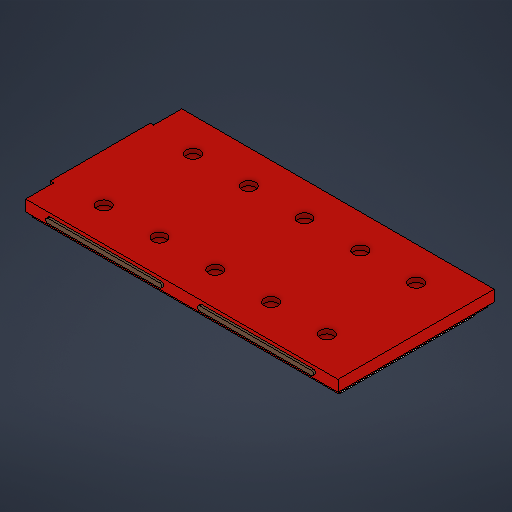
# Autodesk Inventor part: SACMI PH1500 30X60 DIE SET TOP
Saved by Autodesk Inventor 2025 (Build 290162000, 162)
## iProperties
Created: 2024-05-03
Part Number: SACMI PH1500 30X60 DIE SET TOP
Material: Generic
Document SubType Name: Modeling
Designer: zulet
Density: 1 g/cm^3
Appearance: Orange-Red
Author: zulet
Autodesk Inventor part; units mm, degrees
ref_plane "YZ Plane" through (0, 0, 0) normal (1, 0, 0) x (0, 1, 0)
ref_plane "XZ Plane" through (0, 0, 0) normal (0, 1, 0) x (-1, 0, 0)
ref_plane "XY Plane" through (0, 0, 0) normal (0, 0, 1) x (1, 0, 0)
sketch "Sketch1" plane through (0, 0, 0) normal (0, 1, 0) x (-1, 0, 0)
  line L0 (700, 350) -> (-700, 350)
  line L1 (-700, 350) -> (-700, -350)
  line L2 (-700, -350) -> (700, -350)
  line L3 (700, -350) -> (700, 350)
  line L4 (700, 350) -> (-700, -350) construction
  line L5 (-700, 350) -> (700, -350) construction
  point P0 (0, 0)
  dimension "d0" = 1400
  dimension "d1" = 700
  constraints: 12 end point, 2 midpoint, 2 parallel, 1 horizontal, 1 perpendicular
  measures "d0" distance of L2.end L1.end
  measures "d1" distance of L1.end L0.end
extrude "Extrusion1" add sketch "Sketch1" along normal blind 70
sketch "Sketch2" plane through (0, 70, 0) normal (0, 1, 0) x (1, 0, 0)
  line L0 (-500, -200) -> (500, -200) construction
  line L1 (500, -200) -> (500, 200) construction
  line L2 (500, 200) -> (-500, 200) construction
  line L3 (-500, 200) -> (-500, -200) construction
  line L4 (-500, -200) -> (500, 200) construction
  line L5 (500, -200) -> (-500, 200) construction
  circle A0 centre (500, -200) radius 30
  circle A1 centre (250, -200) radius 30
  circle A2 centre (0, -200) radius 30
  circle A3 centre (-250, -200) radius 30
  circle A4 centre (-500, -200) radius 30
  circle A5 centre (500, 200) radius 30
  circle A6 centre (250, 200) radius 30
  circle A7 centre (0, 200) radius 30
  circle A8 centre (-250, 200) radius 30
  circle A9 centre (-500, 200) radius 30
  point P0 (0, 0)
  dimension "d4" = 1000
  dimension "d5" = 400
  dimension "d6" = 60
  dimension "d9" = 250
  dimension "d12" = 400
  constraints: 12 end point, 10 centre point, 2 horizontal, 2 midpoint, 2 parallel, 1 coincident, 1 perpendicular, 1 vertical, 18 other
  measures "d4" distance of L2.end L1.end
  measures "d5" distance of L1.end L0.end
  measures "d6" diameter of A0
  measures "d9" distance of A0.centre A1.centre
  measures "d12" distance of A0.centre A5.centre
extrude "Extrusion2" cut sketch "Sketch2" against normal blind 20
sketch "Sketch3" plane through (0, 0, 0) normal (0, -1, 0) x (1, 0, 0)
  line L0 (700, 350) -> (700, -350) projected
  line L1 (-700, 350) -> (700, 350) projected
  line L2 (-700, -350) -> (-700, 350) projected
  line L3 (700, -350) -> (-700, -350) projected
  line L4 (-685, 335) -> (685, 335)
  line L5 (685, 335) -> (685, -335)
  line L6 (685, -335) -> (-685, -335)
  line L7 (-685, -335) -> (-685, 335)
  point P0 (0, 0)
  dimension "d17" = 15
  constraints: 8 end point, 3 other
  measures "d17" distance between parallel lines of L2 L7
extrude "Extrusion3" cut sketch "Sketch3" against normal blind 20
sketch "Sketch4" plane through (-700, 70, -350) normal (-1, 0, 0) x (0, 0, 1)
  line L0 (125, 0) -> (575, 0)
  line L1 (575, 0) -> (575, -70)
  line L2 (575, -70) -> (125, -70)
  line L3 (125, -70) -> (125, 0)
  line L4 (125, 0) -> (575, -70) construction
  line L5 (575, 0) -> (125, -70) construction
  line L6 (0, 0) -> (700, 0) projected
  line L7 (685, -70) -> (15, -70) projected
  line L8 (350, -35) -> (350, -70) construction
  dimension "d20" = 450
  constraints: 14 end point, 2 collinear, 2 midpoint, 2 parallel, 1 horizontal, 1 perpendicular, 1 vertical
  measures "d20" distance of L0.start L0.end
extrude "Extrusion4" add sketch "Sketch4" along normal blind 15 and the other way blind 15
sketch "Sketch5" plane through (0, 0, 0) normal (0, -1, 0) x (1, 0, 0)
  line L0 (-715, 225) -> (-715, -225) construction
  line L1 (-715, 0) -> (700, 0) construction
  line L2 (700, 350) -> (700, -350) construction
  line L3 (-660, 300) -> (-360, 300) construction
  line L4 (-360, 300) -> (-360, -300) construction
  line L5 (-360, -300) -> (-660, -300) construction
  line L6 (-660, -300) -> (-660, 300) construction
  line L7 (-660, 300) -> (-360, -300) construction
  line L8 (-360, 300) -> (-660, -300) construction
  line L9 (-370, 290) -> (-650, 290)
  line L10 (-650, 290) -> (-650, -290)
  line L11 (-650, -290) -> (-370, -290)
  line L12 (-370, -290) -> (-370, 290)
  line L13 (-320, 300) -> (-20, 300) construction
  line L14 (-20, 300) -> (-20, -300) construction
  line L15 (-20, -300) -> (-320, -300) construction
  line L16 (-320, -300) -> (-320, 300) construction
  line L17 (-320, 300) -> (-20, -300) construction
  line L18 (-20, 300) -> (-320, -300) construction
  line L19 (-30, 290) -> (-310, 290)
  line L20 (-310, 290) -> (-310, -290)
  line L21 (-310, -290) -> (-30, -290)
  line L22 (-30, -290) -> (-30, 290)
  line L23 (20, 300) -> (320, 300) construction
  line L24 (320, 300) -> (320, -300) construction
  line L25 (320, -300) -> (20, -300) construction
  line L26 (20, -300) -> (20, 300) construction
  line L27 (20, 300) -> (320, -300) construction
  line L28 (320, 300) -> (20, -300) construction
  line L29 (310, 290) -> (30, 290)
  line L30 (30, 290) -> (30, -290)
  line L31 (30, -290) -> (310, -290)
  line L32 (310, -290) -> (310, 290)
  line L33 (360, 300) -> (660, 300) construction
  line L34 (660, 300) -> (660, -300) construction
  line L35 (660, -300) -> (360, -300) construction
  line L36 (360, -300) -> (360, 300) construction
  line L37 (360, 300) -> (660, -300) construction
  line L38 (660, 300) -> (360, -300) construction
  line L39 (650, 290) -> (370, 290)
  line L40 (370, 290) -> (370, -290)
  line L41 (370, -290) -> (650, -290)
  line L42 (650, -290) -> (650, 290)
  line L43 (0, 0) -> (0, 331.4551) construction
  point P0 (-510, 0)
  point P1 (-170, 0)
  point P2 (170, 0)
  point P3 (510, 0)
  dimension "d25" = 300
  dimension "d26" = 600
  dimension "d27" = 10
  dimension "d30" = 340
  constraints: 84 end point, 5 parallel, 4 midpoint, 2 horizontal, 2 perpendicular, 1 point on line, 61 other
  measures "d25" distance of L4.end L5.end
  measures "d26" distance of L3.end L4.end
  measures "d27" distance between parallel lines of L3 L9
  measures "d30" distance of L3.start L13.start
extrude "Extrusion5" add sketch "Sketch5" along normal blind 20
sketch "Sketch6" plane through (0, -20, 0) normal (0, -1, 0) x (1, 0, 0)
  line L0 (-650, 290) -> (-650, -290) construction
  line L1 (-650, -290) -> (-370, -290) construction
  line L2 (-370, -290) -> (-370, 290) construction
  line L3 (-370, 290) -> (-650, 290) construction
  line L4 (-310, 290) -> (-310, -290) construction
  line L5 (-310, -290) -> (-30, -290) construction
  line L6 (-30, -290) -> (-30, 290) construction
  line L7 (-30, 290) -> (-310, 290) construction
  line L8 (30, 290) -> (30, -290) construction
  line L9 (30, -290) -> (310, -290) construction
  line L10 (310, -290) -> (310, 290) construction
  line L11 (310, 290) -> (30, 290) construction
  line L12 (370, 290) -> (370, -290) construction
  line L13 (370, -290) -> (650, -290) construction
  line L14 (650, -290) -> (650, 290) construction
  line L15 (650, 290) -> (370, 290) construction
  line L16 (-360, 300) -> (-360, -300)
  line L17 (-360, -300) -> (-660, -300)
  line L18 (-660, -300) -> (-660, 300)
  line L19 (-660, 300) -> (-360, 300)
  line L20 (-320, -300) -> (-320, 300)
  line L21 (-320, 300) -> (-20, 300)
  line L22 (-20, 300) -> (-20, -300)
  line L23 (-20, -300) -> (-320, -300)
  line L24 (20, -300) -> (20, 300)
  line L25 (20, 300) -> (320, 300)
  line L26 (320, 300) -> (320, -300)
  line L27 (320, -300) -> (20, -300)
  line L28 (360, -300) -> (360, 300)
  line L29 (360, 300) -> (660, 300)
  line L30 (660, 300) -> (660, -300)
  line L31 (660, -300) -> (360, -300)
  point P0 (0, 0)
  dimension "d37" = 10
  dimension "d38" = 10
  dimension "d39" = 10
  dimension "d40" = 10
  constraints: 32 end point, 12 other
  measures "d37" distance between parallel lines of L2 L16
  measures "d38" distance between parallel lines of L4 L20
  measures "d39" distance between parallel lines of L8 L24
  measures "d40" distance between parallel lines of L12 L28
extrude "Extrusion6" add sketch "Sketch6" along normal blind 10
sketch "Sketch7" plane through (-650, 0, 290) normal (0, 0, 1) x (1, 0, 0)
  line L0 (280, -20) -> (0, -20) construction
  line L1 (140, -20) -> (140, 0) construction
  line L2 (1335, 0) -> (-35, 0) construction
  circle A0 centre (140, -10) radius 5
  circle A1 centre (480, -10) radius 5
  circle A2 centre (820, -10) radius 5
  circle A3 centre (1160, -10) radius 5
  point P0 (650, 0)
  dimension "d43" = 10
  dimension "d46" = 340
  constraints: 4 centre point, 2 end point, 2 midpoint, 1 horizontal, 1 point on line, 1 vertical, 6 other
  measures "d43" diameter of A0
  measures "d46" distance of A0.centre A1.centre
extrude "Extrusion7" cut sketch "Sketch7" against normal blind 20
sketch "Sketch8" plane through (-370, 0, -290) normal (0, 0, -1) x (-1, 0, 0)
  circle A0 centre (140, -10) radius 5 projected
  circle A1 centre (-200, -10) radius 5 projected
  circle A2 centre (-540, -10) radius 5 projected
  circle A3 centre (-880, -10) radius 5 projected
  point P0 (-370, 0)
extrude "Extrusion8" cut sketch "Sketch8" against normal blind 20
sketch "Sketch9" plane through (-715, 70, -350) normal (-1, 0, 0) x (0, 0, 1)
  line L0 (700, -50) -> (0, -50) projected
  circle A0 centre (180.6783, -50) radius 7.5
  circle A1 centre (259.2358, -18.1737) radius 7.5
  circle A2 centre (358.3679, -32.2018) radius 7.5
  circle A3 centre (497.714, -32.2018) radius 7.5
  circle A4 centre (436.9255, -50) radius 7.5
  circle A5 centre (436.9255, -18.1737) radius 7.5
  point P0 (350, -70)
  dimension "d55" = 15
  dimension "d56" = 15
  dimension "d57" = 15
  dimension "d58" = 15
  dimension "d59" = 15
  dimension "d60" = 15
  constraints: 6 centre point, 2 point on line
  measures "d55" diameter of A0
  measures "d56" diameter of A1
  measures "d57" diameter of A2
  measures "d58" diameter of A3
  measures "d59" diameter of A4
  measures "d60" diameter of A5
extrude "Extrusion9" add sketch "Sketch9" along normal blind 10
sketch "Sketch10" plane through (-700, 70, 350) normal (0, 0, 1) x (1, 0, 0)
  line L0 (0, -50) -> (0, 0) construction
  line L1 (0, -25) -> (1400, -25) construction
  line L2 (1400, -50) -> (1400, 0) construction
  line L3 (110, -25) -> (610, -25) construction
  line L4 (110, -35) -> (610, -35)
  line L5 (610, -15) -> (110, -15)
  arc A0 (110, -15) -> (110, -35) centre (110, -25) ccw
  arc A1 (610, -35) -> (610, -15) centre (610, -25) ccw
  line L6 (700, -70) -> (700, 0) construction
  line L7 (670, 0) -> (730, 0) construction
  line L8 (1290, -35) -> (790, -35)
  line L9 (790, -15) -> (1290, -15)
  arc A2 (1290, -35) -> (1290, -15) centre (1290, -25) ccw
  arc A3 (790, -15) -> (790, -35) centre (790, -25) ccw
  point P0 (360, -25)
  dimension "d63" = 20
  dimension "d64" = 500
  dimension "d65" = 360
  constraints: 16 end point, 8 point on circle, 6 symmetric about line, 4 centre point, 4 midpoint, 4 tangent, 2 point on line, 1 parallel, 2 other
  measures "d63" diameter of A1
  measures "d64" distance of L3.start L3.end
  measures "d65" distance from line of L0 point (360, -25)
extrude "Extrusion10" add sketch "Sketch10" along normal blind 10
equation "\"d9\" = 0.25 * d4"
equation "\"d12\" = d5"
body "Solid1"
